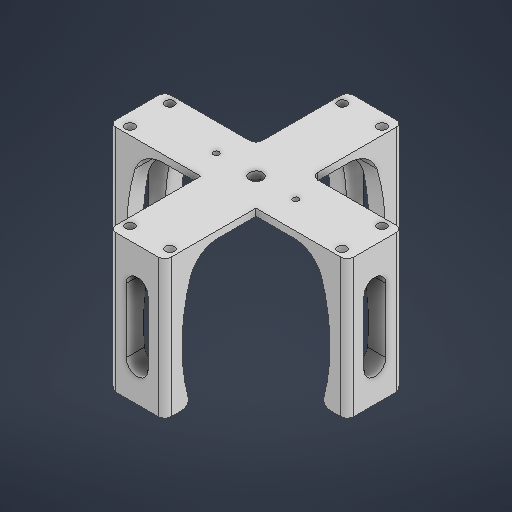
# Autodesk Inventor part: motor_holder
Saved by Autodesk Inventor 2026 (Build 300175050, 175E)
## iProperties
Created: 2025-01-16
Part Number: motor_holder
Material: Generic
Document SubType Name: Modeling
Designer: aduwa
Density: 1 g/cm^3
Appearance: Default
Author: aduwa
Autodesk Inventor part; units mm, degrees
ref_plane "YZ Plane" through (0, 0, 0) normal (1, 0, 0) x (0, 1, 0)
ref_plane "XZ Plane" through (0, 0, 0) normal (0, 1, 0) x (-1, 0, 0)
ref_plane "XY Plane" through (0, 0, 0) normal (0, 0, 1) x (1, 0, 0)
sketch "Sketch1" plane through (0, 0, 0) normal (0, 1, 0) x (1, 0, 0)
  circle A0 centre (0, 0) radius 2.25
  circle A1 centre (31, 0) radius 2.25
  circle A2 centre (0, 31) radius 2.25
  circle A3 centre (31, 31) radius 2.25
  circle A4 centre (15.5, 15.5) radius 5.125
  line L0 (-6, 37) -> (37, 37)
  line L1 (37, 37) -> (37, -6)
  line L2 (37, -6) -> (-6, -6)
  line L3 (-6, -6) -> (-6, 37)
  line L4 (-6, 37) -> (37, -6) construction
  line L5 (37, 37) -> (-6, -6) construction
  line L6 (-6, -6) -> (37, -6)
  circle A5 centre (0, 98) radius 3.5
  circle A6 centre (31, 98) radius 3.5
  line L7 (-6, 37) -> (37, 37)
  line L8 (37, 37) -> (37, 108)
  line L9 (37, 108) -> (-6, 108)
  line L10 (-6, 108) -> (-6, 37)
  line L11 (15.5, 15.5) -> (22.827, 15.5)
  line L12 (-6, 103) -> (37, 103)
  line L13 (-6, 37) -> (-77, 37)
  line L14 (-77, -6) -> (-6, -6)
  circle A7 centre (-67, 0) radius 3.5
  circle A8 centre (-67, 31) radius 3.5
  line L15 (-72, -6) -> (-72, 37)
  line L16 (-77, 37) -> (-77, -6)
  line L17 (-6, -6) -> (-6, -77)
  line L18 (37, -77) -> (37, -6)
  circle A9 centre (31, -67) radius 3.5
  circle A10 centre (0, -67) radius 3.5
  line L19 (37, -72) -> (-6, -72)
  line L20 (-6, -77) -> (37, -77)
  line L21 (37, -6) -> (108, -6)
  line L22 (108, 37) -> (37, 37)
  circle A11 centre (98, 31) radius 3.5
  circle A12 centre (98, 0) radius 3.5
  line L23 (103, 37) -> (103, -6)
  line L24 (108, -6) -> (108, 37)
  line L25 (13, 103) -> (18, 103)
  line L26 (18, 83) -> (13, 83)
  circle A13 centre (-15.5, 15.5) radius 2.25
  circle A14 centre (46.5, 15.5) radius 2.25
  point P0 (37, 37)
  point P1 (37, 37)
  point P2 (-6, -6)
  point P3 (-6, -6)
  point P4 (-6, -6)
  point P5 (-6, -6)
  point P6 (-6, -6)
  point P7 (37, 37)
  point P8 (15.5, 83)
  dimension "d3" = 4.5
  dimension "d5" = 31
  dimension "d6" = 10.25
  dimension "d8" = 43
  dimension "d23" = 7
  dimension "d24" = 31
  dimension "d25" = 31
  dimension "d26" = 82.5
  dimension "d27" = 6
  dimension "d28" = 10
  dimension "d35" = 5
  dimension "d51" = 360
  dimension "d57" = 20
  dimension "d58" = 5
  dimension "d66" = 4.5
  dimension "d67" = 62
  dimension "d68" = 31
  constraints: 54 end point, 15 centre point, 9 point on line, 6 horizontal, 5 equal radius, 5 parallel, 4 horizontal alignment, 4 vertical alignment, 3 midpoint, 2 perpendicular, 1 collinear, 57 other
  measures "d3" diameter of A0
  measures "d5" distance of A0.centre A2.centre
  measures "d6" diameter of A4
  measures "d8" distance of L0.end L1.end
  measures "d23" diameter of A5
  measures "d24" distance of A6.centre A5.centre
  measures "d25" distance of A1.centre A0.centre
  measures "d26" vertical distance of L11.start A6.centre
  measures "d27" distance from line of L0 A2.centre
  measures "d28" distance from line of L9 A5.centre
  measures "d35" distance between parallel lines of L9 L12
  measures "d57" distance of L25.end L26.start
  measures "d58" distance of L26.start L26.end
  measures "d66" diameter of A13
  measures "d67" distance of A14.centre A13.centre
  measures "d68" distance of L11.start A13.centre
extrude "Extrusion4" add sketch "Sketch1" along normal blind 5.5 contours A0 | A1 | A2 | A3 | L10 L12 L8 L0 | L0 L1 L2 L3 | L3 L14 L15 L13 | L22 L23 L21 L1 | L2 L18 L19 L17 | L10 L9 L8 L12 | L15 L14 L16 L13 | L22 L24 L21 L23 | L19 L18 L20 L17
fillet "Fillet4" radius 5 2 edges at (37, 2.75, -37) (-6, 2.75, -37)
fillet "Fillet5" radius 5 8 edges at (37, 2.75, 77) (-6, 2.75, 77) (-77, 2.75, 6) (-77, 2.75, -37) (37, 2.75, -108) (108, 2.75, -37) (108, 2.75, 6) (-6, 2.75, -108)
sketch "Sketch6" plane through (0, 0, 0) normal (0, -1, 0) x (1, 0, 0)
  circle A0 centre (15.5, -15.5) radius 5.125 projected
  line L0 (-11, -37) -> (-72, -37) projected
  line L1 (-77, 6) -> (-57, 6)
  line L2 (-57, 6) -> (-57, -37)
  line L3 (-57, -37) -> (-77, -37)
  line L4 (-77, -37) -> (-77, 6)
  line L5 (-6, -108) -> (-6, -88)
  line L6 (-6, -88) -> (37, -88)
  line L7 (37, -88) -> (37, -108)
  line L8 (37, -108) -> (-6, -108)
  line L9 (108, -37) -> (88, -37)
  line L10 (88, -37) -> (88, 6)
  line L11 (88, 6) -> (108, 6)
  line L12 (108, 6) -> (108, -37)
  line L13 (37, 77) -> (37, 57)
  line L14 (37, 57) -> (-6, 57)
  line L15 (-6, 57) -> (-6, 77)
  line L16 (-6, 77) -> (37, 77)
  circle A1 centre (15.5, -15.5) radius 5.125 projected
  circle A2 centre (31, -98) radius 3.5 projected
  circle A3 centre (0, -98) radius 3.5 projected
  arc A4 (-6, -103) -> (-1, -108) centre (-1, -103) ccw projected
  line L17 (32, -108) -> (-1, -108) projected
  arc A5 (32, -108) -> (37, -103) centre (32, -103) ccw projected
  line L18 (37, -42) -> (37, -103) projected
  arc A6 (42, -37) -> (37, -42) centre (42, -42) ccw projected
  line L19 (103, -37) -> (42, -37) projected
  arc A7 (103, -37) -> (108, -32) centre (103, -32) ccw projected
  line L20 (108, 1) -> (108, -32) projected
  arc A8 (108, 1) -> (103, 6) centre (103, 1) ccw projected
  line L21 (37, 6) -> (103, 6) projected
  line L22 (37, 72) -> (37, 6) projected
  arc A9 (37, 72) -> (32, 77) centre (32, 72) ccw projected
  line L23 (-1, 77) -> (32, 77) projected
  arc A10 (-1, 77) -> (-6, 72) centre (-1, 72) ccw projected
  line L24 (-6, 6) -> (-6, 72) projected
  line L25 (-72, 6) -> (-6, 6) projected
  arc A11 (-72, 6) -> (-77, 1) centre (-72, 1) ccw projected
  line L26 (-77, -32) -> (-77, 1) projected
  arc A12 (-77, -32) -> (-72, -37) centre (-72, -32) ccw projected
  line L27 (-11, -37) -> (-72, -37) projected
  arc A13 (-6, -42) -> (-11, -37) centre (-11, -42) ccw projected
  line L28 (-6, -103) -> (-6, -42) projected
  circle A14 centre (31, 67) radius 3.5 projected
  circle A15 centre (0, 67) radius 3.5 projected
  circle A16 centre (46.5, -15.5) radius 2.25 projected
  circle A17 centre (98, -31) radius 3.5 projected
  circle A18 centre (98, 0) radius 3.5 projected
  circle A19 centre (-67, -31) radius 3.5 projected
  circle A20 centre (-67, 0) radius 3.5 projected
  circle A21 centre (-15.5, -15.5) radius 2.25 projected
  point P0 (0, 0)
  point P1 (98, -31)
  point P2 (31, 67)
  point P3 (-1, -108)
  point P4 (103, 6)
  point P5 (-77, 1)
  point P6 (-6, 72)
  dimension "d71" = 20
  dimension "d74" = 360
  constraints: 32 end point, 2 parallel, 1 horizontal, 1 perpendicular, 1 point on line, 37 other
  measures "d71" distance of L2.end L3.end
extrude "Extrusion7" add sketch "Sketch6" along normal blind 102 contours L0 A12 L4 A11 L1 L2 | L6 L7 A5 L8 A4 L5 | L15 A10 L16 A9 L13 L14 | L10 L11 A8 L12 A7 L9
sketch "Sketch7" plane through (-6, 0, -42) normal (-1, 0, 0) x (0, 0, 1)
  line L0 (-61, 5.5) -> (-61, -102) projected
  line L1 (-46, -102) -> (-61, -102) projected
  line L2 (-46, 0) -> (-46, -102) projected
  line L3 (48, 0) -> (99, 0) projected
  line L4 (0, 5.5) -> (0, 0) projected
  line L5 (-61, 5.5) -> (0, 5.5) projected
  arc A0 (-46, -15) -> (-46, -102) centre (96.3077, -58.5) ccw
  line L6 (-52.5, 5.5) -> (-52.5, -102) projected
  line L7 (114, 5.5) -> (114, -102) projected
  line L8 (48, 5.5) -> (114, 5.5) projected
  line L9 (48, 0) -> (48, 5.5) projected
  line L10 (99, 0) -> (99, -102) projected
  line L11 (114, -102) -> (99, -102) projected
  line L12 (-46, 0) -> (0, 0) projected
  point P0 (42, 0)
  constraints: 2 point on circle, 1 centre point, 1 tangent
extrude "Extrusion8" cut sketch "Sketch7" against normal through all contours A0 L2
pattern_circular "Circular Pattern1" count 4 over 360 about axis through (15.5, 0, -15.5) along (0, 1, 0) of "Extrusion8"
fillet "Fillet8" radius 5 4 edges at (15.5, -102, -88) (88, -102, -15.5) (15.5, -102, 57) (-57, -102, -15.5)
fillet "Fillet9" radius 23 4 edges at (15.5, 0, 57) (88, 0, -15.5) (-57, 0, -15.5) (15.5, 0, -88)
sketch "Sketch8" plane through (32, 5.5, -108) normal (0, 0, -1) x (-1, 0, 0)
  line L0 (16.5, -30.2599) -> (16.5, -80.2599) construction
  line L1 (8, -30.2599) -> (8, -80.2599)
  line L2 (25, -80.2599) -> (25, -30.2599)
  arc A0 (25, -30.2599) -> (8, -30.2599) centre (16.5, -30.2599) ccw
  arc A1 (8, -80.2599) -> (25, -80.2599) centre (16.5, -80.2599) ccw
  line L3 (33, -107.5) -> (0, -107.5) projected
  point P0 (32, -5.5)
  point P1 (16.5, -55.2599)
  point P2 (16.5, -107.5)
  dimension "d86" = 50
  dimension "d87" = 17
  dimension "d88" = 52.2401
  constraints: 8 end point, 4 point on circle, 4 tangent, 2 centre point, 2 midpoint, 1 parallel, 1 vertical, 1 vertical alignment
  measures "d86" distance of L0.start L0.end
  measures "d87" diameter of A1
  measures "d88" distance from line of L3 point (16.5, -55.26)
extrude "Extrusion9" cut sketch "Sketch8" against normal blind 20
pattern_circular "Circular Pattern2" count 4 over 360 about axis through (15.5, 0, -15.5) along (0, 1, 0) of "Extrusion9"
body "Solid2"
